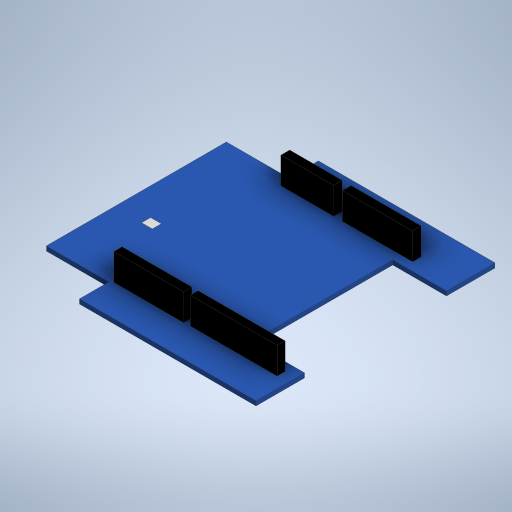
# Autodesk Inventor part: iks01A2base
Saved by Autodesk Inventor 2023 (Build 270158000, 158)
## iProperties
Created: 2023-11-05
Part Number: iks01A2base
Material: Générique
Document SubType Name: Modeling
Designer: eleves
Density: 1 g/cm^3
Appearance: Par défaut
Author: eleves
Autodesk Inventor part; units mm, degrees
ref_plane "YZ Plane" through (0, 0, 0) normal (1, 0, 0) x (0, 1, 0)
ref_plane "XZ Plane" through (0, 0, 0) normal (0, 1, 0) x (-1, 0, 0)
ref_plane "XY Plane" through (0, 0, 0) normal (0, 0, 1) x (1, 0, 0)
sketch "Esquisse1" plane through (0, 0, 0) normal (0, 1, 0) x (-1, 0, 0)
  line L0 (0, 0) -> (78.9893, 0) construction
  line L1 (78.9893, 0) -> (78.9893, -72.281) construction
  line L2 (78.9893, -72.281) -> (0, -72.281) construction
  line L3 (0, -72.281) -> (0, 0) construction
  line L4 (3.8993, -1.7198) -> (2.5066, -1.7198) construction
  line L5 (2.8077, -2.807) -> (2.8077, -1.7198) construction
  line L6 (53.7875, -2.8913) -> (53.7875, -1.7198) construction
  line L7 (53.7875, -1.7198) -> (2.8077, -1.7198) construction
  line L8 (70.571, -10.1894) -> (53.7875, -10.1894) construction
  line L9 (53.7875, -10.1894) -> (53.7875, -1.7198) construction
  line L10 (71.8197, -11.4429) -> (71.8197, -10.1894) construction
  line L11 (71.8197, -10.1894) -> (70.571, -10.1894) construction
  line L12 (71.8197, -10.1894) -> (71.8197, -40.9332) construction
  line L13 (4.0671, -15.7216) -> (2.8077, -15.7216) construction
  line L14 (2.8077, -15.7216) -> (2.8077, -1.7198) construction
  line L15 (4.0671, -15.7216) -> (18.3716, -15.7216) construction
  line L16 (18.326, -19.1106) -> (18.326, -15.7216) construction
  line L17 (18.326, -19.1106) -> (18.326, -45.5089) construction
  line L18 (71.8197, -40.9332) -> (71.8197, -61.0049) construction
  line L19 (70.7314, -62.1766) -> (71.8197, -62.1766) construction
  line L20 (71.8197, -62.1766) -> (71.8197, -61.0049) construction
  line L21 (53.7875, -64.2718) -> (53.7875, -62.1766) construction
  line L22 (53.7875, -62.1766) -> (70.7314, -62.1766) construction
  line L23 (52.6166, -70.7298) -> (53.7875, -70.7298) construction
  line L24 (53.7875, -70.7298) -> (53.7875, -64.2718) construction
  line L25 (16.1382, -56.7226) -> (18.326, -56.7226) construction
  line L26 (18.326, -56.7226) -> (18.326, -45.5089) construction
  line L27 (16.1382, -56.7226) -> (2.8077, -56.7226) construction
  line L28 (52.6166, -70.7298) -> (2.8077, -70.7298) construction
  line L29 (2.8077, -70.7298) -> (2.8077, -56.7226) construction
  line L30 (53.7875, -1.7198) -> (53.7875, -10.1894)
  line L31 (53.7875, -10.1894) -> (71.8197, -10.1894)
  line L32 (71.8197, -10.1894) -> (71.8197, -62.1766)
  line L33 (71.8197, -62.1766) -> (53.7875, -62.1766)
  line L34 (53.7875, -62.1766) -> (53.7875, -70.7298)
  line L35 (53.7875, -70.7298) -> (2.8077, -70.7298)
  line L36 (2.8077, -70.7298) -> (2.8077, -56.7226)
  line L37 (2.8077, -56.7226) -> (18.326, -56.7226)
  line L38 (18.326, -56.7226) -> (18.326, -15.7216)
  line L39 (18.326, -15.7216) -> (2.8077, -15.7216)
  line L40 (2.8077, -15.7216) -> (2.8077, -1.7198)
  line L41 (2.8077, -1.7198) -> (53.7875, -1.7198)
  line L42 (63.8524, -29.7258) -> (60.7561, -29.7258)
  line L43 (60.7561, -29.7258) -> (60.7561, -32.3255)
  line L44 (60.7561, -32.3255) -> (63.8524, -32.3255)
  line L45 (63.8524, -32.3255) -> (63.8524, -29.7258)
  line L46 (5.9145, -13.2045) -> (30.9784, -13.2045)
  line L47 (30.9784, -13.2045) -> (30.9784, -10.944)
  line L48 (30.9784, -10.944) -> (5.9145, -10.944)
  line L49 (5.9145, -10.944) -> (5.9145, -13.2045)
  line L50 (32.8087, -13.2045) -> (52.9636, -13.2045)
  line L51 (52.9636, -13.2045) -> (52.9636, -10.8161)
  line L52 (52.9636, -10.8161) -> (32.8087, -10.8161)
  line L53 (32.8087, -10.8161) -> (32.8087, -13.2045)
  line L54 (37.7726, -59.0838) -> (52.9535, -59.0838)
  line L55 (52.9535, -59.0838) -> (52.9535, -61.5907)
  line L56 (52.9535, -61.5907) -> (37.7726, -61.5907)
  line L57 (37.7726, -61.5907) -> (37.7726, -59.0838)
  line L58 (35.2014, -59.0838) -> (14.9598, -59.0838)
  line L59 (14.9598, -59.0838) -> (14.9598, -61.5907)
  line L60 (14.9598, -61.5907) -> (35.2014, -61.5907)
  line L61 (35.2014, -61.5907) -> (35.2014, -59.0838)
  constraints: 118 end point, 19 perpendicular, 13 parallel, 11 horizontal, 11 point on line, 8 collinear, 3 vertical, 2 other
extrude "Extrusion2" add sketch "Esquisse1" along normal blind 1.3 contours L30 L31 L32 L33 L34 L35 L36 L37 L38 L39 L40 L41 | L45 L44 L43 L42 | L49 L48 L47 L46 | L53 L52 L51 L50 | L54 L55 L56 L57 | L61 L60 L59 L58
extrude "Extrusion3" add sketch "Esquisse1" along normal blind 9 contours L49 L48 L47 L46 | L53 L52 L51 L50 | L54 L55 L56 L57 | L61 L60 L59 L58
extrude "Extrusion4" add sketch "Esquisse1" along normal blind 1.3001 contours L45 L44 L43 L42
sketch "Esquisse2" plane through (0, 0, 0) normal (0, -1, 0) x (1, 0, 0)
  line L0 (-52.9636, -13.2045) -> (-52.9636, -10.8161) projected
  line L1 (-52.9636, -10.8161) -> (-32.8087, -10.8161) projected
  line L2 (-32.8087, -10.8161) -> (-32.8087, -13.2045) projected
  line L3 (-32.8087, -13.2045) -> (-52.9636, -13.2045) projected
  line L4 (-30.9784, -13.2045) -> (-30.9784, -10.944) projected
  line L5 (-30.9784, -10.944) -> (-5.9145, -10.944) projected
  line L6 (-5.9145, -10.944) -> (-5.9145, -13.2045) projected
  line L7 (-5.9145, -13.2045) -> (-30.9784, -13.2045) projected
  line L8 (-37.7726, -61.5907) -> (-52.9535, -61.5907) projected
  line L9 (-52.9535, -61.5907) -> (-52.9535, -59.0838) projected
  line L10 (-52.9535, -59.0838) -> (-37.7726, -59.0838) projected
  line L11 (-37.7726, -59.0838) -> (-37.7726, -61.5907) projected
  line L12 (-14.9598, -59.0838) -> (-14.9598, -61.5907) projected
  line L13 (-14.9598, -61.5907) -> (-35.2014, -61.5907) projected
  line L14 (-35.2014, -61.5907) -> (-35.2014, -59.0838) projected
  line L15 (-35.2014, -59.0838) -> (-14.9598, -59.0838) projected
  line L16 (-5.9145, -12.0742) -> (-52.9636, -12.0103) construction
  circle A0 centre (-7.2085, -12.0725) radius 0.5
  line L17 (-8.4118, -12.0708) -> (-55.4609, -12.0069) construction
  circle A1 centre (-9.7058, -12.0691) radius 0.5
  line L18 (-10.9091, -12.0674) -> (-57.9582, -12.0035) construction
  circle A2 centre (-12.2031, -12.0657) radius 0.5
  line L19 (-13.4064, -12.0641) -> (-60.4555, -12.0001) construction
  circle A3 centre (-14.7004, -12.0623) radius 0.5
  line L20 (-15.9037, -12.0607) -> (-62.9528, -11.9968) construction
  circle A4 centre (-17.1977, -12.0589) radius 0.5
  line L21 (-18.401, -12.0573) -> (-65.4501, -11.9934) construction
  circle A5 centre (-19.695, -12.0555) radius 0.5
  line L22 (-20.8983, -12.0539) -> (-67.9474, -11.99) construction
  circle A6 centre (-22.1923, -12.0521) radius 0.5
  line L23 (-23.3956, -12.0505) -> (-70.4447, -11.9866) construction
  circle A7 centre (-24.6896, -12.0487) radius 0.5
  line L24 (-25.8929, -12.0471) -> (-72.942, -11.9832) construction
  circle A8 centre (-27.1869, -12.0453) radius 0.5
  line L25 (-28.3902, -12.0437) -> (-75.4393, -11.9798) construction
  circle A9 centre (-29.6842, -12.0419) radius 0.5
  circle A10 centre (-34.1027, -12.0359) radius 0.5
  circle A11 centre (-36.5997, -12.0326) radius 0.5
  line L26 (-8.4115, -12.0708) -> (-55.4606, -12.0069) construction
  circle A12 centre (-39.0967, -12.0292) radius 0.5
  line L27 (-10.9085, -12.0674) -> (-57.9576, -12.0035) construction
  circle A13 centre (-41.5937, -12.0258) radius 0.5
  line L28 (-13.4055, -12.0641) -> (-60.4546, -12.0001) construction
  circle A14 centre (-44.0907, -12.0224) radius 0.5
  line L29 (-15.9025, -12.0607) -> (-62.9516, -11.9968) construction
  circle A15 centre (-46.5877, -12.019) radius 0.5
  line L30 (-18.3995, -12.0573) -> (-65.4486, -11.9934) construction
  circle A16 centre (-49.0847, -12.0156) radius 0.5
  line L31 (-20.8965, -12.0539) -> (-67.9456, -11.99) construction
  circle A17 centre (-51.5817, -12.0122) radius 0.5
  line L32 (-23.3935, -12.0505) -> (-70.4426, -11.9866) construction
  line L33 (-14.9598, -60.3373) -> (-52.9535, -60.3373) construction
  circle A18 centre (-16.2538, -60.3373) radius 0.5
  circle A19 centre (-18.7508, -60.3373) radius 0.5
  circle A20 centre (-21.2478, -60.3373) radius 0.5
  circle A21 centre (-23.7448, -60.3373) radius 0.5
  circle A22 centre (-26.2418, -60.3373) radius 0.5
  circle A23 centre (-28.7388, -60.3373) radius 0.5
  circle A24 centre (-31.2358, -60.3373) radius 0.5
  circle A25 centre (-33.7328, -60.3373) radius 0.5
  circle A26 centre (-39.0666, -60.3373) radius 0.5
  circle A27 centre (-41.5636, -60.3373) radius 0.5
  circle A28 centre (-44.0606, -60.3373) radius 0.5
  circle A29 centre (-46.5576, -60.3373) radius 0.5
  circle A30 centre (-49.0546, -60.3373) radius 0.5
  circle A31 centre (-51.5516, -60.3373) radius 0.5
  point P0 (0, 0)
  point P1 (-9.7055, -12.0691)
  point P2 (-12.2025, -12.0657)
  point P3 (-14.6995, -12.0623)
  point P4 (-17.1965, -12.0589)
  point P5 (-19.6935, -12.0555)
  point P6 (-22.1905, -12.0521)
  point P7 (-24.6875, -12.0487)
  dimension "d16" = 1
  dimension "d17" = 1.294
  dimension "d20" = 2.4973
  dimension "d25" = 1
  dimension "d26" = 1.294
  dimension "d29" = 2.497
  dimension "d34" = 1.294
  dimension "d37" = 2.497
  dimension "d42" = 1
  dimension "d43" = 1
  dimension "d44" = 1.294
  dimension "d47" = 2.497
  constraints: 36 end point, 32 centre point, 20 point on line, 4 midpoint, 2 collinear, 2 horizontal, 111 other
  measures "d16" diameter of A0
  measures "d17" distance from line of L6 A0.centre
  measures "d20" distance of L16.start L17.start
  measures "d25" diameter of A10
  measures "d26" distance from line of L2 A10.centre
  measures "d29" distance of A10.centre A11.centre
  measures "d34" distance from line of L12 A18.centre
  measures "d37" distance of A18.centre A19.centre
  measures "d42" diameter of A18
  measures "d43" diameter of A26
  measures "d44" distance from line of L11 A26.centre
  measures "d47" distance of A26.centre A27.centre
extrude "Extrusion5" add sketch "Esquisse2" along normal blind 3 contours A0 | A1 | A2 | A3 | A4 | A5 | A6 | A7 | A8 | A9 | A10 | A11 | A12 | A13 | A14 | A15 | A16 | A17 | A18 | A19 | A20 | A21 | A22 | A23 | A24 | A25 | A26 | A27 | A28 | A29 | A30 | A31
